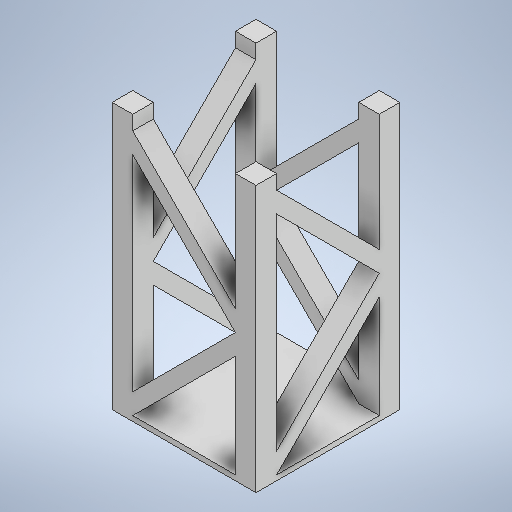
# Autodesk Inventor part: TRUSSTEST
Saved by Autodesk Inventor 2027 (Build 310192060, 192F)
## iProperties
Created: 2026-07-08
Part Number: TRUSSTEST
Material: Generic
Document SubType Name: Modeling
Designer: 13129
Density: 1 g/cm^3
Appearance: Default
Author: 13129
Autodesk Inventor part; units mm, degrees
ref_plane "YZ Plane" through (0, 0, 0) normal (1, 0, 0) x (0, 1, 0)
ref_plane "XZ Plane" through (0, 0, 0) normal (0, 1, 0) x (-1, 0, 0)
ref_plane "XY Plane" through (0, 0, 0) normal (0, 0, 1) x (1, 0, 0)
sketch "Sketch1" plane through (0, 0, 0) normal (0, 1, 0) x (-1, 0, 0)
  line L0 (0, 0) -> (10, 0)
  line L1 (10, 0) -> (10, -10)
  line L2 (10, -10) -> (0, -10)
  line L3 (0, -10) -> (0, 0)
  line L4 (70, -10) -> (60, -10)
  line L5 (60, -10) -> (60, 0)
  line L6 (60, 0) -> (70, 0)
  line L7 (70, 0) -> (70, -10)
  line L8 (70, -70) -> (60, -70)
  line L9 (60, -70) -> (60, -60)
  line L10 (60, -60) -> (70, -60)
  line L11 (70, -60) -> (70, -70)
  line L12 (10, -70) -> (0, -70)
  line L13 (0, -70) -> (0, -60)
  line L14 (0, -60) -> (10, -60)
  line L15 (10, -60) -> (10, -70)
  dimension "d0" = 10
  dimension "d1" = 10
  dimension "d2" = 10
  dimension "d3" = 10
  dimension "d4" = 10
  dimension "d5" = 10
  dimension "d6" = 10
  dimension "d7" = 10
  dimension "d8" = 50
  dimension "d9" = 50
  constraints: 32 end point, 6 parallel, 6 perpendicular, 4 horizontal, 2 horizontal alignment, 2 vertical alignment
  measures "d0" distance of L0.start L0.end
  measures "d1" distance of L0.end L1.end
  measures "d2" distance of L5.end L6.end
  measures "d3" distance of L4.end L5.end
  measures "d4" distance of L9.end L10.end
  measures "d5" distance of L8.end L9.end
  measures "d6" distance of L13.end L14.end
  measures "d7" distance of L12.end L13.end
  measures "d8" distance of L2.end L13.end
  measures "d9" distance of L0.end L5.end
extrude "Extrusion1" add sketch "Sketch1" along normal blind 127
sketch "Sketch2" plane through (-70, 0, 0) normal (0, 0, 1) x (1, 0, 0)
  line L0 (10, 0) -> (10, 127) construction
  line L1 (10, 0) -> (60, 50)
  line L2 (60, 0) -> (60, 127) construction
  line L3 (10, 0) -> (80.7107, 0) construction
  line L4 (10, 10) -> (60, 60)
  line L5 (60, 60) -> (10, 110)
  line L6 (60, 60) -> (130.7107, 60) construction
  line L7 (10, 120) -> (60, 70)
  line L8 (60, 70) -> (60, 50)
  line L9 (10, 120) -> (10, 110)
  line L10 (10, 0) -> (10, 10)
  point P0 (70, 0)
  dimension "d12" = 45
  dimension "d14" = 10
  dimension "d15" = 135
  dimension "d16" = 10
  dimension "d17" = 10
  constraints: 18 end point, 6 point on line, 2 collinear, 2 equal length, 2 horizontal, 1 parallel, 1 vertical
  measures "d12" angle of L3 L1
  measures "d14" distance of L1.end L4.end
  measures "d15" angle of L6 L5
  measures "d16" distance of L4.end L7.end
  measures "d17" distance of L7.start L5.end
extrude "Extrusion2" add sketch "Sketch2" against normal blind 10
sketch "Sketch3" plane through (0, 0, 0) normal (1, 0, 0) x (0, 0, -1)
  line L0 (10, 0) -> (10, 127) construction
  line L1 (10, 0) -> (60, 50)
  line L2 (10, 0) -> (70, 0) construction
  line L3 (60, 0) -> (60, 127) construction
  line L4 (60, 0) -> (70, 0) construction
  line L5 (60, 127) -> (60, 0)
  line L6 (10, 10) -> (60, 60)
  line L7 (10, 0) -> (10, 127)
  line L8 (60, 60) -> (10, 110)
  line L9 (60, 60) -> (70, 60) construction
  line L10 (10, 120) -> (60, 70)
  dimension "d20" = 45
  dimension "d21" = 10
  dimension "d22" = 135
  dimension "d23" = 10
  constraints: 16 end point, 6 point on line, 3 equal length, 2 horizontal, 1 coincident, 1 perpendicular, 1 vertical alignment
  measures "d20" angle of L2 L1
  measures "d21" distance of L0.start L6.start
  measures "d22" angle of L9 L8
  measures "d23" distance of L8.end L10.start
extrude "Extrusion3" add sketch "Sketch3" against normal blind 10 contours L7 L6 L5 L1 | L8 L7 L10 L5
sketch "Sketch4" plane through (0, 0, -70) normal (0, 0, -1) x (-1, 0, 0)
  line L0 (10, 0) -> (10, 127) construction
  line L1 (10, 0) -> (60, 50)
  line L2 (60, 10) -> (60, 110) construction
  line L3 (10, 0) -> (80.7107, 0) construction
  line L4 (10, 10) -> (60, 60)
  line L5 (60, 120) -> (60, 127) construction
  line L6 (60, 127) -> (60, 0)
  line L7 (10, 0) -> (10, 127)
  line L8 (60, 60) -> (10, 110)
  line L9 (60, 60) -> (70, 60) construction
  line L10 (10, 120) -> (60, 70)
  point P0 (70, 0)
  point P1 (60, 60)
  point P2 (60, 60)
  point P3 (60, 50)
  dimension "d26" = 45
  dimension "d27" = 10
  dimension "d28" = 135
  dimension "d29" = 10
  constraints: 16 end point, 6 point on line, 4 equal length, 2 horizontal, 1 midpoint, 1 perpendicular, 1 vertical alignment
  measures "d26" angle of L3 L1
  measures "d27" distance of L4.end L1.end
  measures "d28" angle of L9 L8
  measures "d29" distance of L10.start L8.end
extrude "Extrusion4" add sketch "Sketch4" against normal blind 10 contours L7 L4 L6 L1 | L8 L7 L10 L6
sketch "Sketch5" plane through (-70, 0, -70) normal (-1, 0, 0) x (0, 0, 1)
  line L0 (10, 0) -> (10, 127) construction
  line L1 (60, 10) -> (60, 50) construction
  line L2 (10, 0) -> (60, 50)
  line L3 (10, 0) -> (80.7107, 0) construction
  line L4 (10, 127) -> (10, 0)
  line L5 (60, 127) -> (60, 0)
  line L6 (10, 10) -> (60, 60)
  line L7 (60, 60) -> (10, 110)
  line L8 (60, 60) -> (70, 60) construction
  line L9 (60, 70) -> (10, 120)
  line L10 (10, 70) -> (60, 120) construction
  point P0 (70, 0)
  dimension "d32" = 45
  dimension "d33" = 135
  dimension "d34" = 10
  dimension "d35" = 10
  constraints: 16 end point, 7 point on line, 3 perpendicular, 2 horizontal, 1 coincident, 1 equal length, 1 parallel, 1 vertical alignment
  measures "d32" angle of L3 L2
  measures "d33" angle of L8 L7
  measures "d34" distance of L0.start L6.start
  measures "d35" distance of L6.end L9.start
extrude "Extrusion5" add sketch "Sketch5" against normal blind 10 contours L4 L6 L5 L2 | L7 L4 L9 L5
sketch "Sketch6" plane through (0, 0, 0) normal (0, -1, 0) x (1, 0, 0)
  line L0 (-70, -10) -> (-70, 0) construction
  line L1 (0, -70) -> (-70, -70)
  line L2 (-70, -70) -> (-70, 0)
  line L3 (-70, 0) -> (0, 0)
  line L4 (0, 0) -> (0, -70)
  point P0 (0, 0)
  constraints: 8 end point, 2 parallel, 1 horizontal, 1 perpendicular
extrude "Extrusion6" add sketch "Sketch6" along normal blind 2.5
body "Solid1"
